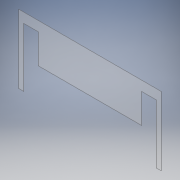
# Autodesk Inventor part: Human Player Ramp Panel
Saved by Autodesk Inventor 2018.3 (Build 223284000, 284)
## iProperties
Created: 2020-03-05
Part Number: Human Player Ramp Panel
Material: Polycarbonate, Clear
Document SubType Name: Modeling
Designer: carls
Mass: 356.419 g
Surface Area: 3773.38 cm^2
Volume: 297.016 cm^3
Density: 1.2 g/cm^3
Appearance: Polycarbonate - Clear
Author: carls
Autodesk Inventor part; units mm, degrees
ref_plane "YZ Plane" through (0, 0, 0) normal (1, 0, 0) x (0, 1, 0)
ref_plane "XZ Plane" through (0, 0, 0) normal (0, 1, 0) x (-1, 0, 0)
ref_plane "XY Plane" through (0, 0, 0) normal (0, 0, 1) x (1, 0, 0)
sketch "Sketch1" plane through (0, 0, 0) normal (0, 0, 1) x (1, 0, 0)
  line L0 (-368.3, -177.8) -> (368.3, -177.8)
  line L1 (368.3, -177.8) -> (368.3, 177.8)
  line L2 (368.3, 177.8) -> (-368.3, 177.8)
  line L3 (-368.3, 177.8) -> (-368.3, -177.8)
  line L4 (-368.3, -177.8) -> (368.3, 177.8) construction
  line L5 (368.3, -177.8) -> (-368.3, 177.8) construction
  point P0 (0, 0)
  dimension "d0" = 355.6
  dimension "d1" = 736.6
  constraints: 12 end point, 2 midpoint, 2 parallel, 1 horizontal, 1 perpendicular
  measures "d0" distance of L2.end L0.start
  measures "d1" distance of L1.end L2.end
extrude "Extrusion1" add sketch "Sketch1" along normal blind 1.5875
sketch "Sketch2" plane through (0, 0, 1.5875) normal (0, 0, 1) x (1, 0, 0)
  line L0 (-368.3, -177.8) -> (368.3, -177.8) projected
  line L1 (368.3, -177.8) -> (368.3, 177.8) projected
  line L2 (368.3, 177.8) -> (-368.3, 177.8) projected
  line L3 (-368.3, 177.8) -> (-368.3, -177.8) projected
  line L4 (-368.3, -177.8) -> (368.3, -177.8) projected
  line L5 (-342.9, -177.8) -> (-266.7, -177.8)
  line L6 (-266.7, -177.8) -> (-266.7, 127)
  line L7 (-266.7, 127) -> (-342.9, 127)
  line L8 (-342.9, 127) -> (-342.9, -177.8)
  point P0 (0, 0)
  dimension "d4" = 50.8
  dimension "d5" = 76.2
  dimension "d6" = 25.4
  constraints: 8 end point, 2 parallel, 1 horizontal, 1 perpendicular, 1 point on line
  measures "d4" distance between parallel lines of L2 L7
  measures "d5" distance between parallel lines of L6 L8
  measures "d6" distance between parallel lines of L8 L3
extrude "Extrusion2" cut sketch "Sketch2" against normal through all contours L8 L7 L6 L0
mirror "Mirror1" about plane through (0, 0, 0) normal (1, 0, 0) of "Extrusion2"
sketch "Sketch3" plane through (0, 0, 1.5875) normal (0, 0, 1) x (1, 0, 0)
  line L0 (342.9, 127) -> (342.9, -177.8) projected
  line L1 (342.9, -177.8) -> (368.3, -177.8) projected
  line L2 (368.3, -177.8) -> (368.3, 177.8) projected
  line L3 (368.3, 177.8) -> (-368.3, 177.8) projected
  line L4 (-368.3, 177.8) -> (-368.3, -177.8) projected
  line L5 (-368.3, -177.8) -> (-342.9, -177.8) projected
  line L6 (-342.9, -177.8) -> (-342.9, 127) projected
  line L7 (-342.9, 127) -> (-266.7, 127) projected
  line L8 (-266.7, 127) -> (-266.7, -177.8) projected
  line L9 (-266.7, -177.8) -> (266.7, -177.8) projected
  line L10 (266.7, -177.8) -> (266.7, 127) projected
  line L11 (266.7, 127) -> (342.9, 127) projected
  line L12 (-266.7, -177.8) -> (266.7, -177.8)
  line L13 (266.7, -177.8) -> (266.7, -25.4)
  line L14 (266.7, -25.4) -> (-266.7, -25.4)
  line L15 (-266.7, -25.4) -> (-266.7, -177.8)
  point P0 (0, 0)
  dimension "d9" = 152.4
  constraints: 8 end point, 2 parallel, 1 collinear, 1 horizontal, 1 perpendicular
  measures "d9" distance between parallel lines of L5 L14
extrude "Extrusion3" cut sketch "Sketch3" against normal through all contours L10 L9 L8 L14
body "Solid1"
